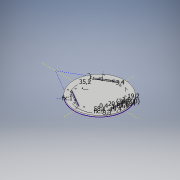
# Autodesk Inventor part: Stewart-Platform-Base-Innenanordnung
Saved by Autodesk Inventor 2018.2 (Build 222227000, 227)
## iProperties
Created: 2018-02-17
Part Number: Stewart-Platform-Base-Innenanordnung
Material: Generisch
Document SubType Name: Modeling
Designer: JochenAlt
Density: 1 g/cm^3
Appearance: Vorgabe
Author: JochenAlt
Autodesk Inventor part; units mm, degrees
ref_plane "YZ Plane" through (0, 0, 0) normal (1, 0, 0) x (0, 1, 0)
ref_plane "XZ Plane" through (0, 0, 0) normal (0, 1, 0) x (-1, 0, 0)
ref_plane "XY Plane" through (0, 0, 0) normal (0, 0, 1) x (1, 0, 0)
sketch "Skizze1" plane through (0, 0, 0) normal (0, 0, 1) x (1, 0, 0)
  line L0 (0, 78.2107) -> (0, -78.2107) construction
  line L1 (-128.6657, 0) -> (86.6199, 0) construction
  line L2 (31.7553, 29.05) -> (44.1553, 29.05) construction
  line L3 (47.5553, 25.65) -> (47.5553, -25.65) construction
  line L4 (44.1553, -29.05) -> (31.7553, -29.05) construction
  line L5 (28.3553, -25.65) -> (28.3553, 25.65) construction
  arc A0 (31.7553, 29.05) -> (28.3553, 25.65) centre (31.7553, 25.65) ccw construction
  arc A1 (47.5553, 25.65) -> (44.1553, 29.05) centre (44.1553, 25.65) ccw construction
  arc A2 (44.1553, -29.05) -> (47.5553, -25.65) centre (44.1553, -25.65) ccw construction
  arc A3 (28.3553, -25.65) -> (31.7553, -29.05) centre (31.7553, -25.65) ccw construction
  circle A4 centre (31.7553, 25.65) radius 1.4
  circle A5 centre (44.1553, 25.65) radius 1.4
  circle A6 centre (31.7553, -25.65) radius 1.4
  circle A7 centre (44.1553, -25.65) radius 1.4
  line L6 (41.6553, 21.4) -> (41.6553, -21.4)
  line L7 (38.3553, 21.4) -> (38.3553, -21.4)
  line L8 (38.3553, 21.4) -> (41.6553, 21.4)
  line L9 (38.3553, -21.4) -> (41.6553, -21.4)
  line L10 (38.3553, 0.8) -> (41.6553, 0.8)
  line L11 (38.3553, -0.8) -> (41.6553, -0.8)
  line L12 (41.6553, 12.5) -> (44.5713, 12.5)
  line L13 (44.5713, 12.5) -> (44.5713, 9.7)
  line L14 (44.5713, 9.7) -> (41.6553, 9.7)
  line L15 (41.6553, -9.7) -> (44.5713, -9.7)
  line L16 (44.5713, -9.7) -> (44.5713, -12.5)
  line L17 (44.5713, -12.5) -> (41.6553, -12.5)
  line L18 (44.1553, 29.45) -> (31.7553, 29.45)
  arc A8 (31.7553, 29.45) -> (27.9553, 25.65) centre (31.7553, 25.65) ccw
  line L19 (27.9553, 25.65) -> (27.9553, -25.65)
  arc A9 (27.9553, -25.65) -> (31.7553, -29.45) centre (31.7553, -25.65) ccw
  line L20 (31.7553, -29.45) -> (44.1553, -29.45)
  arc A10 (44.1553, -29.45) -> (47.9553, -25.65) centre (44.1553, -25.65) ccw
  line L21 (47.9553, -25.65) -> (47.9553, 25.65)
  arc A11 (47.9553, 25.65) -> (44.1553, 29.45) centre (44.1553, 25.65) ccw
  line L22 (25.9072, -29.1198) -> (28.4872, -27.589) construction
  line L23 (-0.6447, 43.9167) -> (-2.2947, 46.7745)
  circle A12 centre (0.1359, 51.0646) radius 1.4
  arc A13 (3.0804, 52.7646) -> (-1.5641, 54.0091) centre (0.1359, 51.0646) ccw construction
  arc A14 (3.4268, 52.9646) -> (-1.7641, 54.3555) centre (0.1359, 51.0646) ccw
  circle A15 centre (6.3359, 40.3259) radius 1.4
  line L24 (12.2649, 36.9962) -> (9.6492, 38.4652) construction
  arc A16 (8.0359, 37.3814) -> (9.2804, 42.0259) centre (6.3359, 40.3259) ccw construction
  arc A17 (8.2359, 37.035) -> (9.6268, 42.2259) centre (6.3359, 40.3259) ccw
  line L25 (9.6268, 42.2259) -> (3.4268, 52.9646)
  line L26 (3.0804, 52.7646) -> (9.2804, 42.0259) construction
  line L27 (-41.0357, 12.9759) -> (-47.2357, 23.7146) construction
  arc A18 (-41.0357, 12.9759) -> (-36.3912, 11.7314) centre (-38.0912, 14.6759) ccw construction
  circle A19 centre (-38.0912, 14.6759) radius 1.4
  circle A20 centre (-44.2912, 25.4146) radius 1.4
  arc A21 (-41.3821, 12.7759) -> (-36.1912, 11.385) centre (-38.0912, 14.6759) ccw
  line L28 (-47.5821, 23.5146) -> (-41.3821, 12.7759)
  arc A22 (-45.9912, 28.3591) -> (-47.2357, 23.7146) centre (-44.2912, 25.4146) ccw construction
  arc A23 (-46.1912, 28.7055) -> (-47.5821, 23.5146) centre (-44.2912, 25.4146) ccw
  line L29 (-11.4603, 44.8499) -> (-10.0023, 42.3245)
  line L30 (-13.8852, 43.4499) -> (-11.4603, 44.8499)
  line L31 (-12.4272, 40.9245) -> (-13.8852, 43.4499)
  line L32 (-37.7106, 22.5167) -> (-39.3606, 25.3745)
  line L33 (-31.653, 29.8245) -> (-33.111, 32.3499)
  line L34 (-33.111, 32.3499) -> (-30.6861, 33.7499)
  line L35 (-30.6861, 33.7499) -> (-29.2281, 31.2245)
  line L36 (-19.8705, 32.8167) -> (-21.5205, 35.6745)
  line L37 (-18.4848, 33.6167) -> (-20.1348, 36.4745)
  line L38 (-39.3606, 25.3745) -> (-2.2947, 46.7745)
  line L39 (-1.7641, 54.3555) -> (-46.1912, 28.7055)
  line L40 (-45.9912, 28.3591) -> (-1.5641, 54.0091) construction
  line L41 (8.0359, 37.3814) -> (-36.3912, 11.7314) construction
  line L42 (-36.1912, 11.385) -> (8.2359, 37.035)
  line L43 (-37.7106, 22.5167) -> (-0.6447, 43.9167)
  line L44 (-37.7106, -22.5167) -> (-39.3606, -25.3745)
  circle A24 centre (-44.2912, -25.4146) radius 1.4
  arc A25 (-47.2357, -23.7146) -> (-45.9912, -28.3591) centre (-44.2912, -25.4146) ccw construction
  arc A26 (-47.5821, -23.5146) -> (-46.1912, -28.7055) centre (-44.2912, -25.4146) ccw
  circle A27 centre (-38.0912, -14.6759) radius 1.4
  line L45 (-38.1721, -7.8764) -> (-38.1364, -10.8762) construction
  arc A28 (-36.3912, -11.7314) -> (-41.0357, -12.9759) centre (-38.0912, -14.6759) ccw construction
  arc A29 (-36.1912, -11.385) -> (-41.3821, -12.7759) centre (-38.0912, -14.6759) ccw
  line L46 (-41.3821, -12.7759) -> (-47.5821, -23.5146)
  line L47 (-47.2357, -23.7146) -> (-41.0357, -12.9759) construction
  line L48 (9.2804, -42.0259) -> (3.0804, -52.7646) construction
  arc A30 (9.2804, -42.0259) -> (8.0359, -37.3814) centre (6.3359, -40.3259) ccw construction
  circle A31 centre (6.3359, -40.3259) radius 1.4
  circle A32 centre (0.1359, -51.0646) radius 1.4
  arc A33 (9.6268, -42.2259) -> (8.2359, -37.035) centre (6.3359, -40.3259) ccw
  line L49 (3.4268, -52.9646) -> (9.6268, -42.2259)
  arc A34 (-1.5641, -54.0091) -> (3.0804, -52.7646) centre (0.1359, -51.0646) ccw construction
  arc A35 (-1.7641, -54.3555) -> (3.4268, -52.9646) centre (0.1359, -51.0646) ccw
  line L50 (-33.111, -32.3499) -> (-31.653, -29.8245)
  line L51 (-30.6861, -33.7499) -> (-33.111, -32.3499)
  line L52 (-29.2281, -31.2245) -> (-30.6861, -33.7499)
  line L53 (-0.6447, -43.9167) -> (-2.2947, -46.7745)
  line L54 (-10.0023, -42.3245) -> (-11.4603, -44.8499)
  line L55 (-11.4603, -44.8499) -> (-13.8852, -43.4499)
  line L56 (-13.8852, -43.4499) -> (-12.4272, -40.9245)
  line L57 (-18.4848, -33.6167) -> (-20.1348, -36.4745)
  line L58 (-19.8705, -32.8167) -> (-21.5205, -35.6745)
  line L59 (-2.2947, -46.7745) -> (-39.3606, -25.3745)
  line L60 (-46.1912, -28.7055) -> (-1.7641, -54.3555)
  line L61 (-1.5641, -54.0091) -> (-45.9912, -28.3591) construction
  line L62 (-36.3912, -11.7314) -> (8.0359, -37.3814) construction
  line L63 (8.2359, -37.035) -> (-36.1912, -11.385)
  line L64 (-0.6447, -43.9167) -> (-37.7106, -22.5167)
  line L65 (-31.8985, 33.0499) -> (-43.6029, 53.3224) construction
  line L66 (-34.0905, 36.8465) -> (-97.9106, 0) construction
  line L67 (-31.8985, -33.0499) -> (-43.7977, -53.6598) construction
  line L68 (-34.0905, -36.8465) -> (-97.9106, 0) construction
  circle A36 centre (0, 0) radius 55.8648
  line L69 (-48.4545, 27.8035) -> (-47.5871, 27.3058) construction
  line L70 (-42.3106, 30.4841) -> (-24.7106, 0) construction
  dimension "d1" = 58.1
  dimension "d2" = 19.2
  dimension "d3" = 3.4
  dimension "d5" = 2.8
  dimension "d6" = 5.9
  dimension "d7" = 3.3
  dimension "d8" = 20.6
  dimension "d9" = 1.6
  dimension "d10" = 2.984
  dimension "d11" = 2.8
  dimension "d12" = 19.4
  dimension "d21" = 0.4
  dimension "d22" = 3
  dimension "d32" = 360
  dimension "d44" = 1
  dimension "d45" = 1
  dimension "d47" = 1
  dimension "d53" = 35.2
  constraints: 138 end point, 52 point on circle, 36 centre point, 30 point on line, 13 coincident, 10 perpendicular, 8 tangent, 6 equal radius, 6 horizontal, 6 parallel, 2 collinear, 2 line through centre, 2 midpoint, 2 vertical, 242 other
  measures "d1" distance between parallel lines of L4 L2
  measures "d2" distance between parallel lines of L3 L5
  measures "d3" radius of A0
  measures "d5" diameter of A4
  measures "d6" distance between parallel lines of L3 L6
  measures "d7" distance between parallel lines of L6 L7
  measures "d8" distance between parallel lines of L10 L8
  measures "d9" distance between parallel lines of L11 L10
  measures "d10" distance between parallel lines of L3 L13
  measures "d11" distance between parallel lines of L14 L12
  measures "d12" distance between parallel lines of L15 L14
  measures "d21" distance between parallel lines of L19 L5
  measures "d22" distance of L22.end L22.start
  measures "d44" distance between parallel lines of L39 L66
  measures "d45" distance between parallel lines of L68 L60
  measures "d47" distance of L69.start L69.end
  measures "d53" distance of L70.start L70.end
extrude "Extrusion5" add sketch "Skizze1" along normal blind 3 contours A11 L21 A10 L20 A9 L19 A8 L18 | L25 A17 L42 A21 L28 A23 L39 A14 | L46 A29 L63 A33 L49 A35 L60 A26 | A36
extrude "Extrusion4" cut sketch "Skizze1" along normal blind 1 contours L10 L6 L11 L7 | A11 L21 A10 L20 A9 L19 A8 L18 | L43 L36 L38 L37 | L25 A17 L42 A21 L28 A23 L39 A14 | L64 L57 L59 L58 | L46 A29 L63 A33 L49 A35 L60 A26
equation "\"d22\" = d20"
equation "\"d20\" = 3"
